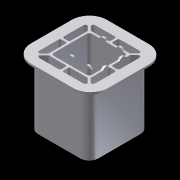
# Autodesk Inventor part: Part4
Saved by Autodesk Inventor 2012 (Build 160160000, 160)
## iProperties
Created: 2012-10-11
Part Number: Part4
Material: Default
Document SubType Name: Modeling
Designer: SONY
Density: 1 g/cm^3
Author: SONY
Autodesk Inventor part; units mm, degrees
ref_plane "YZ Plane" through (0, 0, 0) normal (1, 0, 0) x (0, 1, 0)
ref_plane "XZ Plane" through (0, 0, 0) normal (0, 1, 0) x (-1, 0, 0)
ref_plane "XY Plane" through (0, 0, 0) normal (0, 0, 1) x (1, 0, 0)
sketch "Sketch1" plane through (0, 0, 0) normal (0, 0, 1) x (1, 0, 0)
  line L0 (-50.8, 30.4821) -> (-50.8, -23.4929) projected
  arc A0 (-50.8, -23.4929) -> (-47.625, -26.6679) centre (-47.625, -23.4929) ccw projected
  line L1 (-47.625, -26.6679) -> (47.625, -26.6679) projected
  arc A1 (47.625, -26.6679) -> (50.8, -23.4929) centre (47.625, -23.4929) ccw projected
  line L2 (50.8, -23.4929) -> (50.8, 30.4821) projected
  line L3 (50.8, 30.4821) -> (25.4, 30.4821) projected
  line L4 (25.4, 30.4821) -> (25.4, 1.9071) projected
  arc A2 (22.225, -1.2679) -> (25.4, 1.9071) centre (22.225, 1.9071) ccw projected
  line L5 (22.225, -1.2679) -> (-22.225, -1.2679) projected
  arc A3 (-25.4, 1.9071) -> (-22.225, -1.2679) centre (-22.225, 1.9071) ccw projected
  line L6 (-25.4, 1.9071) -> (-25.4, 30.4821) projected
  line L7 (-25.4, 30.4821) -> (-50.8, 30.4821) projected
  arc A4 (-47.625, 87.6321) -> (-50.8, 84.4571) centre (-47.625, 84.4571) ccw projected
  line L8 (-50.8, 30.4821) -> (-50.8, 84.4571) projected
  line L9 (-25.4, 30.4821) -> (-50.8, 30.4821) projected
  line L10 (-25.4, 59.0571) -> (-25.4, 30.4821) projected
  arc A5 (-22.225, 62.2321) -> (-25.4, 59.0571) centre (-22.225, 59.0571) ccw projected
  line L11 (22.225, 62.2321) -> (-22.225, 62.2321) projected
  arc A6 (25.4, 59.0571) -> (22.225, 62.2321) centre (22.225, 59.0571) ccw projected
  line L12 (25.4, 30.4821) -> (25.4, 59.0571) projected
  line L13 (50.8, 30.4821) -> (25.4, 30.4821) projected
  line L14 (50.8, 84.4571) -> (50.8, 30.4821) projected
  arc A7 (50.8, 84.4571) -> (47.625, 87.6321) centre (47.625, 84.4571) ccw projected
  line L15 (-47.625, 87.6321) -> (47.625, 87.6321) projected
  line L16 (21.015, 0.6371) -> (19.215, 0.6371)
  line L17 (19.215, 0.6371) -> (19.215, 60.3271)
  line L18 (19.215, 60.3271) -> (21.015, 60.3271)
  line L19 (21.015, 60.3271) -> (21.015, 0.6371)
  line L20 (55.185, 0.6371) -> (56.985, 0.6371)
  line L21 (56.985, 0.6371) -> (56.985, 60.3271)
  line L22 (56.985, 60.3271) -> (55.185, 60.3271)
  line L23 (55.185, 60.3271) -> (55.185, 0.6371)
  line L24 (25.1349, 0.6371) -> (23.0176, 0.6371)
  line L25 (25.1349, 60.3271) -> (25.3032, 60.3271)
  line L26 (26.765, 60.3271) -> (23.1302, 60.3271) projected
  line L27 (23.015, 60.3271) -> (23.015, 0.6371) projected
  line L28 (53.185, -14.6029) -> (53.185, 64.1371) projected
  point P0 (0, 0)
  dimension "d0" = 1.8
  dimension "d1" = 1.8
  dimension "d34" = 59.69
  dimension "d115" = 2
  dimension "d116" = 2
  constraints: 20 end point, 4 collinear, 4 horizontal, 4 parallel, 2 perpendicular, 2 point on circle, 3 other
  measures "d0" distance between parallel lines of L23 L21
  measures "d1" distance of L17.end L18.end
  measures "d34" distance of L20.end L21.end
  measures "d115" distance between parallel lines of L27 L19
  measures "d116" distance between parallel lines of L23 L28
extrude "center_a" add sketch "Sketch1" against normal blind 25.4 contours L16 L17 L18 L19 | L23 L22 L21 L20
sketch "Sketch2" plane through (0, 0, 0) normal (0, 0, 1) x (1, 0, 0)
  line L0 (55.185, 0.6371) -> (56.985, 0.6371) projected
  line L1 (56.985, 0.6371) -> (56.985, 60.3271) projected
  line L2 (56.985, 60.3271) -> (55.185, 60.3271) projected
  line L3 (55.185, 60.3271) -> (55.185, 0.6371) projected
  line L4 (21.015, 0.6371) -> (19.215, 0.6371) projected
  line L5 (21.015, 60.3271) -> (21.015, 0.6371) projected
  line L6 (19.215, 60.3271) -> (21.015, 60.3271) projected
  line L7 (19.215, 0.6371) -> (19.215, 60.3271) projected
  arc A0 (-47.625, 87.6321) -> (-50.8, 84.4571) centre (-47.625, 84.4571) ccw projected
  line L8 (-50.8, 30.4821) -> (-50.8, 84.4571) projected
  line L9 (-25.4, 30.4821) -> (-50.8, 30.4821) projected
  line L10 (-25.4, 59.0571) -> (-25.4, 30.4821) projected
  arc A1 (-22.225, 62.2321) -> (-25.4, 59.0571) centre (-22.225, 59.0571) ccw projected
  line L11 (22.225, 62.2321) -> (-22.225, 62.2321) projected
  arc A2 (25.4, 59.0571) -> (22.225, 62.2321) centre (22.225, 59.0571) ccw projected
  line L12 (25.4, 30.4821) -> (25.4, 59.0571) projected
  line L13 (50.8, 30.4821) -> (25.4, 30.4821) projected
  line L14 (50.8, 84.4571) -> (50.8, 30.4821) projected
  arc A3 (50.8, 84.4571) -> (47.625, 87.6321) centre (47.625, 84.4571) ccw projected
  line L15 (-47.625, 87.6321) -> (47.625, 87.6321) projected
  line L16 (-50.8, 30.4821) -> (-50.8, -23.4929) projected
  arc A4 (-50.8, -23.4929) -> (-47.625, -26.6679) centre (-47.625, -23.4929) ccw projected
  line L17 (-47.625, -26.6679) -> (47.625, -26.6679) projected
  arc A5 (47.625, -26.6679) -> (50.8, -23.4929) centre (47.625, -23.4929) ccw projected
  line L18 (50.8, -23.4929) -> (50.8, 30.4821) projected
  line L19 (50.8, 30.4821) -> (25.4, 30.4821) projected
  line L20 (25.4, 30.4821) -> (25.4, 1.9071) projected
  arc A6 (22.225, -1.2679) -> (25.4, 1.9071) centre (22.225, 1.9071) ccw projected
  line L21 (22.225, -1.2679) -> (-22.225, -1.2679) projected
  arc A7 (-25.4, 1.9071) -> (-22.225, -1.2679) centre (-22.225, 1.9071) ccw projected
  line L22 (-25.4, 1.9071) -> (-25.4, 30.4821) projected
  line L23 (-25.4, 30.4821) -> (-50.8, 30.4821) projected
  point P0 (0, 0)
extrude "center_b" add sketch "Sketch2" along normal blind 4.4525 contours L3 L2 L1 L0 | L4 L7 L6 L5
sketch "Sketch3" plane through (0, 0, -25.4) normal (0, 0, -1) x (-1, 0, 0)
  line L0 (-21.015, 0.6371) -> (-21.015, 60.3271) projected
  line L1 (-19.215, 0.6371) -> (-21.015, 0.6371) projected
  line L2 (-19.215, 60.3271) -> (-19.215, 0.6371) projected
  line L3 (-21.015, 60.3271) -> (-19.215, 60.3271) projected
  line L4 (-56.985, 0.6371) -> (-56.985, 60.3271) projected
  line L5 (-55.185, 0.6371) -> (-56.985, 0.6371) projected
  line L6 (-55.185, 60.3271) -> (-55.185, 0.6371) projected
  line L7 (-56.985, 60.3271) -> (-55.185, 60.3271) projected
  point P0 (0, 0)
extrude "center_c" add sketch "Sketch3" along normal blind 4.4525
sketch "Sketch4" plane through (0, 0, -29.8525) normal (0, 0, -1) x (-1, 0, 0)
  line L0 (-56.985, 60.3271) -> (-55.185, 60.3271) projected
  line L1 (-56.985, 0.6371) -> (-56.985, 60.3271) projected
  line L2 (-55.185, 0.6371) -> (-56.985, 0.6371) projected
  line L3 (-55.185, 60.3271) -> (-55.185, 0.6371) projected
  line L4 (-56.985, 60.3271) -> (-19.215, 60.3271)
  line L5 (-19.215, 60.3271) -> (-19.215, 0.6371)
  line L6 (-19.215, 0.6371) -> (-56.985, 0.6371)
  line L7 (-56.985, 0.6371) -> (-56.985, 60.3271)
  point P0 (0, 0)
  constraints: 8 end point, 2 parallel, 1 horizontal, 1 perpendicular
extrude "center_d" add sketch "Sketch4" along normal blind 1.8
sketch "Sketch5" plane through (0, 0, 4.4525) normal (0, 0, 1) x (1, 0, 0)
  line L0 (55.185, 0.6371) -> (55.185, 60.3271) projected
  line L1 (56.985, 0.6371) -> (55.185, 0.6371) projected
  line L2 (56.985, 60.3271) -> (56.985, 0.6371) projected
  line L3 (55.185, 60.3271) -> (56.985, 60.3271) projected
  line L4 (19.215, 60.3271) -> (56.985, 60.3271)
  line L5 (56.985, 60.3271) -> (56.985, 0.6371)
  line L6 (56.985, 0.6371) -> (19.215, 0.6371)
  line L7 (19.215, 0.6371) -> (19.215, 60.3271)
  point P0 (0, 0)
  constraints: 8 end point, 2 parallel, 1 horizontal, 1 perpendicular
extrude "center_e" add sketch "Sketch5" along normal blind 1.8
fillet "internal-fillet" radius 3 4 edges at (19.215, 30.4821, -31.6525) (56.985, 30.4821, -31.6525) (19.215, 30.4821, 6.2525) (56.985, 30.4821, 6.2525)
fillet "internal-fillet" radius 2.5 4 edges at (55.185, 30.4821, -29.8525) (55.185, 30.4821, 4.4525) (21.015, 30.4821, 4.4525) (21.015, 30.4821, -29.8525)
sketch "Sketch25" plane through (22.215, 0.6371, 6.2525) normal (0, -1, 0) x (1, 0, 0)
  arc A0 (34.77, -3) -> (31.77, 0) centre (31.77, -3) ccw projected
  line L0 (31.77, 0) -> (0, 0) projected
  arc A1 (0, 0) -> (-3, -3) centre (0, -3) ccw projected
  line L1 (-3, -3) -> (-3, -34.905) projected
  arc A2 (-3, -34.905) -> (0, -37.905) centre (0, -34.905) ccw projected
  line L2 (0, -37.905) -> (31.77, -37.905) projected
  arc A3 (31.77, -37.905) -> (34.77, -34.905) centre (31.77, -34.905) ccw projected
  line L3 (34.77, -34.905) -> (34.77, -3) projected
  line L4 (1.3, -1.8) -> (30.47, -1.8) projected
  line L5 (-3, 8.15) -> (34.77, 8.15)
  line L6 (42.92, 0) -> (42.92, -37.905)
  line L7 (34.77, -46.055) -> (-3, -46.055)
  line L8 (-11.15, -37.905) -> (-11.15, 0)
  line L9 (-3, 0) -> (34.77, 0) construction
  line L10 (34.77, 0) -> (34.77, -37.905) construction
  line L11 (34.77, -37.905) -> (-3, -37.905) construction
  line L12 (-3, -37.905) -> (-3, 0) construction
  arc A4 (-3, 8.15) -> (-11.15, 0) centre (-3, 0) ccw
  arc A5 (-11.15, -37.905) -> (-3, -46.055) centre (-3, -37.905) ccw
  arc A6 (34.77, -46.055) -> (42.92, -37.905) centre (34.77, -37.905) ccw
  arc A7 (42.92, 0) -> (34.77, 8.15) centre (34.77, 0) ccw
  line L13 (34.77, 0) -> (-3, -37.905) construction
  line L14 (34.77, -37.905) -> (-3, 0) construction
  line L15 (16.5203, -18.315) -> (-8.0799, 6.3731) construction
  line L16 (15.2497, -19.59) -> (-9.355, 5.1026) construction
  line L17 (15.2497, -19.59) -> (39.8499, -44.2781) construction
  line L18 (16.5203, -18.315) -> (41.125, -43.0076) construction
  line L19 (-9.355, -43.0076) -> (39.8499, 6.3731) construction
  line L20 (41.125, 5.1026) -> (-8.0799, -44.2781) construction
  line L21 (39.8444, -41.7225) -> (34.4312, -36.2899)
  line L22 (38.5693, -42.993) -> (33.1595, -37.5638)
  line L23 (-6.7993, -42.993) -> (-1.3895, -37.5638)
  line L24 (-8.0744, -41.7225) -> (-2.6612, -36.2899)
  line L25 (-2.6612, -1.6151) -> (-8.0744, 3.8175)
  line L26 (-6.7993, 5.088) -> (-1.3895, -0.3412)
  line L27 (33.1595, -0.3412) -> (38.5693, 5.088)
  line L28 (39.8444, 3.8175) -> (34.4312, -1.6151)
  line L29 (15.885, -18.9525) -> (55.6698, -18.9525) construction
  line L30 (15.885, -18.9525) -> (-18.4202, -18.9525) construction
  line L31 (15.885, -18.9525) -> (15.885, 6.5335) construction
  line L32 (15.885, -18.9525) -> (15.885, -60.1449) construction
  line L33 (14.985, 22.3974) -> (16.785, 22.3974) construction
  line L34 (16.785, 22.3974) -> (16.785, -69.4541) construction
  line L35 (16.785, -69.4541) -> (14.985, -69.4541) construction
  line L36 (14.985, -69.4541) -> (14.985, 22.3974) construction
  line L37 (64.878, -19.8525) -> (-35.3195, -19.8525) construction
  line L38 (-35.3195, -19.8525) -> (-35.3195, -18.0525) construction
  line L39 (-35.3195, -18.0525) -> (64.878, -18.0525) construction
  line L40 (64.878, -18.0525) -> (64.878, -19.8525) construction
  line L41 (34.77, -18.0525) -> (41.12, -18.0525)
  line L42 (41.12, -19.8525) -> (34.77, -19.8525)
  line L43 (16.785, 0) -> (16.785, 6.35)
  line L44 (14.985, 6.35) -> (14.985, 0)
  line L45 (-3, -18.0525) -> (-9.35, -18.0525)
  line L46 (-9.35, -19.8525) -> (-3, -19.8525)
  line L47 (16.785, -37.905) -> (16.785, -44.255)
  line L48 (14.985, -44.255) -> (14.985, -37.905)
  line L49 (41.12, 0) -> (41.12, -18.0525)
  line L50 (41.12, -19.8525) -> (41.12, -37.905)
  line L51 (-9.35, -37.905) -> (-9.35, -19.8525)
  line L52 (-9.35, -18.0525) -> (-9.35, 0)
  line L53 (34.77, -44.255) -> (16.785, -44.255)
  line L54 (14.985, -44.255) -> (-3, -44.255)
  arc A8 (34.77, -44.255) -> (38.5693, -42.993) centre (34.77, -37.905) ccw
  arc A9 (39.8444, -41.7225) -> (41.12, -37.905) centre (34.77, -37.905) ccw
  arc A10 (-9.35, -37.905) -> (-8.0744, -41.7225) centre (-3, -37.905) ccw
  arc A11 (-6.7993, -42.993) -> (-3, -44.255) centre (-3, -37.905) ccw
  arc A12 (41.12, 0) -> (39.8444, 3.8175) centre (34.77, 0) ccw
  arc A13 (38.5693, 5.088) -> (34.77, 6.35) centre (34.77, 0) ccw
  line L55 (-3, 6.35) -> (14.985, 6.35)
  line L56 (16.785, 6.35) -> (34.77, 6.35)
  arc A14 (-3, 6.35) -> (-6.7993, 5.088) centre (-3, 0) ccw
  arc A15 (-8.0744, 3.8175) -> (-9.35, 0) centre (-3, 0) ccw
  line L57 (-3, -18.0525) -> (-3, -19.8525)
  line L58 (14.985, 0) -> (16.785, 0)
  line L59 (34.77, -18.0525) -> (34.77, -19.8525)
  line L60 (16.785, -37.905) -> (14.985, -37.905)
  line L61 (19.3458, 41.1317) -> (44.9845, 41.1317) construction
  line L62 (44.9845, 41.1317) -> (44.9845, 37.9997) construction
  line L63 (44.9845, 37.9997) -> (19.3458, 37.9997) construction
  line L64 (19.3458, 37.9997) -> (19.3458, 41.1317) construction
  dimension "d166" = 1.8
  dimension "d171" = 0.9
  dimension "d172" = 1.8
  dimension "d173" = 1.8
  dimension "d174" = 0.9
  dimension "d175" = 0.9
  dimension "d176" = 0.9
  dimension "d177" = 0.9
  dimension "d178" = 1.8
  dimension "d179" = 1.8
  dimension "d180" = 1.8
  dimension "d181" = 6.35
  dimension "d182" = 6.35
  dimension "d183" = 6.35
  constraints: 112 end point, 42 point on line, 40 point on circle, 23 parallel, 22 tangent, 12 centre point, 10 collinear, 10 perpendicular, 8 coincident, 6 horizontal, 1 midpoint, 2 other
  measures "d166" distance between parallel lines of L4 L0
  measures "d171" distance between parallel lines of L15 L14
  measures "d172" distance between parallel lines of L16 L15
  measures "d173" distance between parallel lines of L19 L20
  measures "d174" distance between parallel lines of L13 L19
  measures "d175" distance between parallel lines of L32 L36
  measures "d176" distance between parallel lines of L32 L34
  measures "d177" distance between parallel lines of L29 L37
  measures "d178" distance between parallel lines of L37 L39
  measures "d179" radial gap between concentric circles of A5 A10
  measures "d180" distance between parallel lines of L54 L7
  measures "d181" distance between parallel lines of L55 L0
  measures "d182" distance between parallel lines of L1 L52
  measures "d183" distance between parallel lines of L49 L3
extrude "spiderweb" add sketch "Sketch25" against normal up to surface (59.69 mm away)
sketch "Sketch26" plane through (19.215, 60.3271, 14.4025) normal (0, 1, 0) x (1, 0, 0)
  line L0 (0, -8.8849) -> (37.77, -8.8849)
  line L1 (56.08, 9.4251) -> (56.08, 46.055)
  line L2 (37.77, 64.365) -> (0, 64.365)
  line L3 (-18.31, 46.055) -> (-18.31, 9.4251)
  arc A0 (-18.31, 9.4251) -> (0, -8.8849) centre (0, 9.4251) ccw
  arc A1 (37.77, -8.8849) -> (56.08, 9.4251) centre (37.77, 9.4251) ccw
  arc A2 (56.08, 46.055) -> (37.77, 64.365) centre (37.77, 46.055) ccw
  arc A3 (0, 64.365) -> (-18.31, 46.055) centre (0, 46.055) ccw
  arc A4 (37.4312, 9.7651) -> (37.77, 11.15) centre (34.77, 11.15) ccw projected
  line L4 (37.77, 26.2025) -> (37.77, 11.15) projected
  line L5 (44.12, 26.2025) -> (37.77, 26.2025) projected
  line L6 (44.12, 8.15) -> (44.12, 26.2025) projected
  arc A5 (42.8444, 4.3325) -> (44.12, 8.15) centre (37.77, 8.15) ccw projected
  line L7 (37.4312, 9.7651) -> (42.8444, 4.3325) projected
  line L8 (37.77, 43.055) -> (37.77, 28.0025) projected
  arc A6 (37.77, 43.055) -> (37.4312, 44.4399) centre (34.77, 43.055) ccw projected
  line L9 (42.8444, 49.8725) -> (37.4312, 44.4399) projected
  arc A7 (44.12, 46.055) -> (42.8444, 49.8725) centre (37.77, 46.055) ccw projected
  line L10 (44.12, 28.0025) -> (44.12, 46.055) projected
  line L11 (37.77, 28.0025) -> (44.12, 28.0025) projected
  arc A8 (36.1595, 45.7138) -> (34.77, 46.055) centre (34.77, 43.055) ccw projected
  line L12 (34.77, 46.055) -> (19.785, 46.055) projected
  line L13 (19.785, 52.405) -> (19.785, 46.055) projected
  line L14 (37.77, 52.405) -> (19.785, 52.405) projected
  arc A9 (41.5693, 51.143) -> (37.77, 52.405) centre (37.77, 46.055) ccw projected
  line L15 (36.1595, 45.7138) -> (41.5693, 51.143) projected
  line L16 (17.985, 46.055) -> (3, 46.055) projected
  arc A10 (3, 46.055) -> (1.6105, 45.7138) centre (3, 43.055) ccw projected
  line L17 (-3.7993, 51.143) -> (1.6105, 45.7138) projected
  arc A11 (0, 52.405) -> (-3.7993, 51.143) centre (0, 46.055) ccw projected
  line L18 (17.985, 52.405) -> (0, 52.405) projected
  line L19 (17.985, 46.055) -> (17.985, 52.405) projected
  line L20 (0, 11.15) -> (0, 26.2025) projected
  arc A12 (0, 11.15) -> (0.3388, 9.7651) centre (3, 11.15) ccw projected
  line L21 (-5.0744, 4.3325) -> (0.3388, 9.7651) projected
  arc A13 (-6.35, 8.15) -> (-5.0744, 4.3325) centre (0, 8.15) ccw projected
  line L22 (-6.35, 26.2025) -> (-6.35, 8.15) projected
  line L23 (0, 26.2025) -> (-6.35, 26.2025) projected
  line L24 (-6.35, 28.0025) -> (0, 28.0025) projected
  line L25 (-6.35, 46.055) -> (-6.35, 28.0025) projected
  arc A14 (-5.0744, 49.8725) -> (-6.35, 46.055) centre (0, 46.055) ccw projected
  line L26 (0.3388, 44.4399) -> (-5.0744, 49.8725) projected
  arc A15 (0.3388, 44.4399) -> (0, 43.055) centre (3, 43.055) ccw projected
  line L27 (0, 28.0025) -> (0, 43.055) projected
  arc A16 (1.6105, 8.4912) -> (3, 8.15) centre (3, 11.15) ccw projected
  line L28 (3, 8.15) -> (17.985, 8.15) projected
  line L29 (17.985, 1.8) -> (17.985, 8.15) projected
  line L30 (0, 1.8) -> (17.985, 1.8) projected
  arc A17 (-3.7993, 3.062) -> (0, 1.8) centre (0, 8.15) ccw projected
  line L31 (1.6105, 8.4912) -> (-3.7993, 3.062) projected
  arc A18 (-8.15, 8.15) -> (0, 0) centre (0, 8.15) ccw projected
  line L32 (37.77, 0) -> (0, 0) projected
  arc A19 (37.77, 0) -> (45.92, 8.15) centre (37.77, 8.15) ccw projected
  line L33 (45.92, 46.055) -> (45.92, 8.15) projected
  arc A20 (45.92, 46.055) -> (37.77, 54.205) centre (37.77, 46.055) ccw projected
  line L34 (0, 54.205) -> (37.77, 54.205) projected
  arc A21 (0, 54.205) -> (-8.15, 46.055) centre (0, 46.055) ccw projected
  line L35 (-8.15, 8.15) -> (-8.15, 46.055) projected
  line L36 (41.5693, 3.062) -> (36.1595, 8.4912) projected
  arc A22 (37.77, 1.8) -> (41.5693, 3.062) centre (37.77, 8.15) ccw projected
  line L37 (19.785, 1.8) -> (37.77, 1.8) projected
  line L38 (19.785, 8.15) -> (19.785, 1.8) projected
  line L39 (19.785, 8.15) -> (34.77, 8.15) projected
  arc A23 (34.77, 8.15) -> (36.1595, 8.4912) centre (34.77, 11.15) ccw projected
  line L40 (33.47, 9.95) -> (4.3, 9.95) projected
  arc A24 (1.8, 12.45) -> (4.3, 9.95) centre (4.3, 12.45) ccw projected
  line L41 (1.8, 12.45) -> (1.8, 41.755) projected
  arc A25 (4.3, 44.255) -> (1.8, 41.755) centre (4.3, 41.755) ccw projected
  line L42 (4.3, 44.255) -> (33.47, 44.255) projected
  arc A26 (35.97, 41.755) -> (33.47, 44.255) centre (33.47, 41.755) ccw projected
  line L43 (35.97, 41.755) -> (35.97, 12.45) projected
  arc A27 (33.47, 9.95) -> (35.97, 12.45) centre (33.47, 12.45) ccw projected
  dimension "d206" = 10.16
  constraints: 8 end point, 8 point on circle, 8 tangent, 4 centre point, 3 perpendicular, 2 coincident, 2 horizontal alignment, 2 vertical alignment, 1 point on line
  measures "d206" distance between parallel lines of L2 L34
extrude "flat base" add sketch "Sketch26" against normal blind 1.8 contours A0 L3 A3 L2 A2 L1 A1 L0
fillet "superfillet" radius 1.5 40 edges at (60.7843, 30.4821, 11.3405) (62.0594, 30.4821, 10.07) (63.335, 30.4821, -11.8) (63.335, 30.4821, -13.6) (62.0594, 30.4821, -35.47) (60.7843, 30.4821, -36.7405) (39, 30.4821, -38.0025) (37.2, 30.4821, -38.0025) (14.1406, 30.4821, 10.07) (12.865, 30.4821, -11.8) (12.865, 30.4821, -13.6) (14.1406, 30.4821, -35.47) (39, 30.4821, 12.6025) (37.2, 30.4821, 12.6025) (15.4157, 30.4821, 11.3405) (15.4157, 30.4821, -36.7405) (19.215, 30.4821, -11.8) (20.8255, 30.4821, 5.9113) (55.3745, 30.4821, 5.9113) (56.985, 30.4821, -11.8) (56.6462, 30.4821, 4.6374) (39, 30.4821, 6.2525) (19.215, 30.4821, -13.6) (20.8255, 30.4821, -31.3113) (19.5538, 30.4821, -30.0374) (39, 30.4821, -31.6525) (37.2, 30.4821, -31.6525) (56.6462, 30.4821, -30.0374) (56.985, 30.4821, -13.6) (55.3745, 30.4821, -31.3113) (13.4521, 58.5271, 12.0154) (11.065, 58.5271, -12.7) (13.4521, 58.5271, -37.4154) (38.1, 58.5271, -39.8025) (62.7479, 58.5271, -37.4154) (65.135, 58.5271, -12.7) (62.7479, 58.5271, 12.0154) (38.1, 58.5271, 14.4025) (37.2, 30.4821, 6.2525) (19.5538, 30.4821, 4.6374)
sketch "Sketch27" plane through (19.215, 0.6371, 14.4025) normal (0, -1, 0) x (1, 0, 0)
  arc A0 (35.4337, -8.2243) -> (34.77, -8.15) centre (34.77, -11.15) ccw projected
  line L0 (34.77, -8.15) -> (21.285, -8.15) projected
  arc A1 (19.785, -6.65) -> (21.285, -8.15) centre (21.285, -6.65) ccw projected
  line L1 (19.785, -6.65) -> (19.785, -3.3) projected
  arc A2 (21.285, -1.8) -> (19.785, -3.3) centre (21.285, -3.3) ccw projected
  line L2 (21.285, -1.8) -> (37.77, -1.8) projected
  arc A3 (39.439, -2.0233) -> (37.77, -1.8) centre (37.77, -8.15) ccw projected
  arc A4 (40.1073, -4.5293) -> (39.439, -2.0233) centre (39.0447, -3.4705) ccw projected
  line L3 (40.1073, -4.5293) -> (36.828, -7.8203) projected
  arc A5 (35.4337, -8.2243) -> (36.828, -7.8203) centre (35.7655, -6.7615) ccw projected
  line L4 (38.0964, -9.0975) -> (41.3824, -5.7998) projected
  arc A6 (43.8907, -6.4592) -> (41.3824, -5.7998) centre (42.4449, -6.8586) ccw projected
  arc A7 (44.12, -8.15) -> (43.8907, -6.4592) centre (37.77, -8.15) ccw projected
  line L5 (44.12, -8.15) -> (44.12, -24.7025) projected
  arc A8 (42.62, -26.2025) -> (44.12, -24.7025) centre (42.62, -24.7025) ccw projected
  line L6 (42.62, -26.2025) -> (39.27, -26.2025) projected
  arc A9 (37.77, -24.7025) -> (39.27, -26.2025) centre (39.27, -24.7025) ccw projected
  line L7 (37.77, -24.7025) -> (37.77, -11.15) projected
  arc A10 (37.77, -11.15) -> (37.6959, -10.4875) centre (34.77, -11.15) ccw projected
  arc A11 (38.0964, -9.0975) -> (37.6959, -10.4875) centre (39.1589, -10.1563) ccw projected
  line L8 (39.27, -28.0025) -> (42.62, -28.0025) projected
  arc A12 (44.12, -29.5025) -> (42.62, -28.0025) centre (42.62, -29.5025) ccw projected
  line L9 (44.12, -29.5025) -> (44.12, -46.055) projected
  arc A13 (43.8907, -47.7458) -> (44.12, -46.055) centre (37.77, -46.055) ccw projected
  arc A14 (41.3824, -48.4052) -> (43.8907, -47.7458) centre (42.4449, -47.3464) ccw projected
  line L10 (41.3824, -48.4052) -> (38.0964, -45.1075) projected
  arc A15 (37.6959, -43.7175) -> (38.0964, -45.1075) centre (39.1589, -44.0487) ccw projected
  arc A16 (37.6959, -43.7175) -> (37.77, -43.055) centre (34.77, -43.055) ccw projected
  line L11 (37.77, -43.055) -> (37.77, -29.5025) projected
  arc A17 (39.27, -28.0025) -> (37.77, -29.5025) centre (39.27, -29.5025) ccw projected
  line L12 (36.828, -46.3847) -> (40.1073, -49.6757) projected
  arc A18 (39.439, -52.1817) -> (40.1073, -49.6757) centre (39.0447, -50.7345) ccw projected
  arc A19 (37.77, -52.405) -> (39.439, -52.1817) centre (37.77, -46.055) ccw projected
  line L13 (37.77, -52.405) -> (21.285, -52.405) projected
  arc A20 (19.785, -50.905) -> (21.285, -52.405) centre (21.285, -50.905) ccw projected
  line L14 (19.785, -50.905) -> (19.785, -47.555) projected
  arc A21 (21.285, -46.055) -> (19.785, -47.555) centre (21.285, -47.555) ccw projected
  line L15 (21.285, -46.055) -> (34.77, -46.055) projected
  arc A22 (34.77, -46.055) -> (35.4337, -45.9807) centre (34.77, -43.055) ccw projected
  arc A23 (36.828, -46.3847) -> (35.4337, -45.9807) centre (35.7655, -47.4435) ccw projected
  line L16 (0, -29.5025) -> (0, -43.055) projected
  arc A24 (0, -43.055) -> (0.0741, -43.7175) centre (3, -43.055) ccw projected
  arc A25 (-0.3264, -45.1075) -> (0.0741, -43.7175) centre (-1.3889, -44.0487) ccw projected
  line L17 (-0.3264, -45.1075) -> (-3.6124, -48.4052) projected
  arc A26 (-6.1207, -47.7458) -> (-3.6124, -48.4052) centre (-4.6749, -47.3464) ccw projected
  arc A27 (-6.35, -46.055) -> (-6.1207, -47.7458) centre (0, -46.055) ccw projected
  line L18 (-6.35, -46.055) -> (-6.35, -29.5025) projected
  arc A28 (-4.85, -28.0025) -> (-6.35, -29.5025) centre (-4.85, -29.5025) ccw projected
  line L19 (-4.85, -28.0025) -> (-1.5, -28.0025) projected
  arc A29 (0, -29.5025) -> (-1.5, -28.0025) centre (-1.5, -29.5025) ccw projected
  line L20 (17.985, -47.555) -> (17.985, -50.905) projected
  arc A30 (16.485, -52.405) -> (17.985, -50.905) centre (16.485, -50.905) ccw projected
  line L21 (16.485, -52.405) -> (0, -52.405) projected
  arc A31 (-1.669, -52.1817) -> (0, -52.405) centre (0, -46.055) ccw projected
  arc A32 (-2.3373, -49.6757) -> (-1.669, -52.1817) centre (-1.2747, -50.7345) ccw projected
  line L22 (-2.3373, -49.6757) -> (0.942, -46.3847) projected
  arc A33 (2.3363, -45.9807) -> (0.942, -46.3847) centre (2.0045, -47.4435) ccw projected
  arc A34 (2.3363, -45.9807) -> (3, -46.055) centre (3, -43.055) ccw projected
  line L23 (3, -46.055) -> (16.485, -46.055) projected
  arc A35 (17.985, -47.555) -> (16.485, -46.055) centre (16.485, -47.555) ccw projected
  line L24 (0, 0) -> (37.77, 0) projected
  arc A36 (0, 0) -> (-8.15, -8.15) centre (0, -8.15) ccw projected
  line L25 (-8.15, -46.055) -> (-8.15, -8.15) projected
  arc A37 (-8.15, -46.055) -> (0, -54.205) centre (0, -46.055) ccw projected
  line L26 (37.77, -54.205) -> (0, -54.205) projected
  arc A38 (37.77, -54.205) -> (45.92, -46.055) centre (37.77, -46.055) ccw projected
  line L27 (45.92, -8.15) -> (45.92, -46.055) projected
  arc A39 (45.92, -8.15) -> (37.77, 0) centre (37.77, -8.15) ccw projected
  line L28 (35.97, -12.45) -> (35.97, -41.755) projected
  arc A40 (33.47, -44.255) -> (35.97, -41.755) centre (33.47, -41.755) ccw projected
  line L29 (33.47, -44.255) -> (4.3, -44.255) projected
  arc A41 (1.8, -41.755) -> (4.3, -44.255) centre (4.3, -41.755) ccw projected
  line L30 (1.8, -41.755) -> (1.8, -12.45) projected
  arc A42 (4.3, -9.95) -> (1.8, -12.45) centre (4.3, -12.45) ccw projected
  line L31 (4.3, -9.95) -> (33.47, -9.95) projected
  arc A43 (35.97, -12.45) -> (33.47, -9.95) centre (33.47, -12.45) ccw projected
  arc A44 (35.4337, -8.2243) -> (34.77, -8.15) centre (34.77, -11.15) ccw projected
  line L32 (34.77, -8.15) -> (21.285, -8.15) projected
  arc A45 (19.785, -6.65) -> (21.285, -8.15) centre (21.285, -6.65) ccw projected
  line L33 (19.785, -6.65) -> (19.785, -3.3) projected
  line L34 (40.1073, -4.5293) -> (36.828, -7.8203) projected
  arc A46 (35.4337, -8.2243) -> (36.828, -7.8203) centre (35.7655, -6.7615) ccw projected
  line L35 (38.0964, -9.0975) -> (41.3824, -5.7998) projected
  line L36 (42.62, -26.2025) -> (39.27, -26.2025) projected
  arc A47 (37.77, -24.7025) -> (39.27, -26.2025) centre (39.27, -24.7025) ccw projected
  line L37 (37.77, -24.7025) -> (37.77, -11.15) projected
  arc A48 (37.77, -11.15) -> (37.6959, -10.4875) centre (34.77, -11.15) ccw projected
  arc A49 (38.0964, -9.0975) -> (37.6959, -10.4875) centre (39.1589, -10.1563) ccw projected
  line L38 (39.27, -28.0025) -> (42.62, -28.0025) projected
  line L39 (41.3824, -48.4052) -> (38.0964, -45.1075) projected
  arc A50 (37.6959, -43.7175) -> (38.0964, -45.1075) centre (39.1589, -44.0487) ccw projected
  arc A51 (37.6959, -43.7175) -> (37.77, -43.055) centre (34.77, -43.055) ccw projected
  line L40 (37.77, -43.055) -> (37.77, -29.5025) projected
  arc A52 (39.27, -28.0025) -> (37.77, -29.5025) centre (39.27, -29.5025) ccw projected
  line L41 (36.828, -46.3847) -> (40.1073, -49.6757) projected
  arc A53 (39.439, -52.1817) -> (40.1073, -49.6757) centre (39.0447, -50.7345) ccw projected
  arc A54 (37.77, -52.405) -> (39.439, -52.1817) centre (37.77, -46.055) ccw projected
  line L42 (37.77, -52.405) -> (21.285, -52.405) projected
  arc A55 (19.785, -50.905) -> (21.285, -52.405) centre (21.285, -50.905) ccw projected
  line L43 (19.785, -50.905) -> (19.785, -47.555) projected
  arc A56 (21.285, -46.055) -> (19.785, -47.555) centre (21.285, -47.555) ccw projected
  line L44 (21.285, -46.055) -> (34.77, -46.055) projected
  arc A57 (34.77, -46.055) -> (35.4337, -45.9807) centre (34.77, -43.055) ccw projected
  arc A58 (36.828, -46.3847) -> (35.4337, -45.9807) centre (35.7655, -47.4435) ccw projected
  line L45 (0, -29.5025) -> (0, -43.055) projected
  arc A59 (0, -43.055) -> (0.0741, -43.7175) centre (3, -43.055) ccw projected
  arc A60 (-0.3264, -45.1075) -> (0.0741, -43.7175) centre (-1.3889, -44.0487) ccw projected
  line L46 (-0.3264, -45.1075) -> (-3.6124, -48.4052) projected
  arc A61 (-6.1207, -47.7458) -> (-3.6124, -48.4052) centre (-4.6749, -47.3464) ccw projected
  arc A62 (-6.35, -46.055) -> (-6.1207, -47.7458) centre (0, -46.055) ccw projected
  line L47 (-6.35, -46.055) -> (-6.35, -29.5025) projected
  arc A63 (-4.85, -28.0025) -> (-6.35, -29.5025) centre (-4.85, -29.5025) ccw projected
  line L48 (-4.85, -28.0025) -> (-1.5, -28.0025) projected
  arc A64 (0, -29.5025) -> (-1.5, -28.0025) centre (-1.5, -29.5025) ccw projected
  line L49 (17.985, -47.555) -> (17.985, -50.905) projected
  arc A65 (16.485, -52.405) -> (17.985, -50.905) centre (16.485, -50.905) ccw projected
  line L50 (16.485, -52.405) -> (0, -52.405) projected
  arc A66 (-1.669, -52.1817) -> (0, -52.405) centre (0, -46.055) ccw projected
  arc A67 (-2.3373, -49.6757) -> (-1.669, -52.1817) centre (-1.2747, -50.7345) ccw projected
  line L51 (-2.3373, -49.6757) -> (0.942, -46.3847) projected
  arc A68 (2.3363, -45.9807) -> (0.942, -46.3847) centre (2.0045, -47.4435) ccw projected
  arc A69 (2.3363, -45.9807) -> (3, -46.055) centre (3, -43.055) ccw projected
  line L52 (3, -46.055) -> (16.485, -46.055) projected
  arc A70 (17.985, -47.555) -> (16.485, -46.055) centre (16.485, -47.555) ccw projected
  line L53 (-1.5, -26.2025) -> (-4.85, -26.2025) projected
  arc A71 (-6.35, -24.7025) -> (-4.85, -26.2025) centre (-4.85, -24.7025) ccw projected
  line L54 (-6.35, -24.7025) -> (-6.35, -8.15) projected
  arc A72 (-6.1207, -6.4592) -> (-6.35, -8.15) centre (0, -8.15) ccw projected
  arc A73 (-3.6124, -5.7998) -> (-6.1207, -6.4592) centre (-4.6749, -6.8586) ccw projected
  line L55 (-3.6124, -5.7998) -> (-0.3264, -9.0975) projected
  arc A74 (0.0741, -10.4875) -> (-0.3264, -9.0975) centre (-1.3889, -10.1563) ccw projected
  arc A75 (0.0741, -10.4875) -> (0, -11.15) centre (3, -11.15) ccw projected
  line L56 (0, -11.15) -> (0, -24.7025) projected
  arc A76 (-1.5, -26.2025) -> (0, -24.7025) centre (-1.5, -24.7025) ccw projected
  line L57 (0, 0) -> (37.77, 0) projected
  arc A77 (0, 0) -> (-8.15, -8.15) centre (0, -8.15) ccw projected
  line L58 (-8.15, -46.055) -> (-8.15, -8.15) projected
  arc A78 (-8.15, -46.055) -> (0, -54.205) centre (0, -46.055) ccw projected
  line L59 (37.77, -54.205) -> (0, -54.205) projected
  arc A79 (37.77, -54.205) -> (45.92, -46.055) centre (37.77, -46.055) ccw projected
  line L60 (45.92, -8.15) -> (45.92, -46.055) projected
  arc A80 (45.92, -8.15) -> (37.77, 0) centre (37.77, -8.15) ccw projected
  line L61 (0.942, -7.8203) -> (-2.3373, -4.5293) projected
  line L62 (17.985, -3.3) -> (17.985, -6.65) projected
  arc A81 (16.485, -8.15) -> (17.985, -6.65) centre (16.485, -6.65) ccw projected
  line L63 (16.485, -8.15) -> (3, -8.15) projected
  arc A82 (3, -8.15) -> (2.3363, -8.2243) centre (3, -11.15) ccw projected
  arc A83 (0.942, -7.8203) -> (2.3363, -8.2243) centre (2.0045, -6.7615) ccw projected
  line L64 (35.97, -12.45) -> (35.97, -41.755) projected
  arc A84 (33.47, -44.255) -> (35.97, -41.755) centre (33.47, -41.755) ccw projected
  line L65 (33.47, -44.255) -> (4.3, -44.255) projected
  arc A85 (1.8, -41.755) -> (4.3, -44.255) centre (4.3, -41.755) ccw projected
  line L66 (1.8, -41.755) -> (1.8, -12.45) projected
  arc A86 (4.3, -9.95) -> (1.8, -12.45) centre (4.3, -12.45) ccw projected
  line L67 (4.3, -9.95) -> (33.47, -9.95) projected
  arc A87 (35.97, -12.45) -> (33.47, -9.95) centre (33.47, -12.45) ccw projected
  arc A88 (21.285, -1.8) -> (19.785, -3.3) centre (21.285, -3.3) ccw projected
  line L68 (21.285, -1.8) -> (37.77, -1.8) projected
  arc A89 (39.439, -2.0233) -> (37.77, -1.8) centre (37.77, -8.15) ccw projected
  arc A90 (40.1073, -4.5293) -> (39.439, -2.0233) centre (39.0447, -3.4705) ccw projected
  arc A91 (43.8907, -6.4592) -> (41.3824, -5.7998) centre (42.4449, -6.8586) ccw projected
  arc A92 (44.12, -8.15) -> (43.8907, -6.4592) centre (37.77, -8.15) ccw projected
  line L69 (44.12, -8.15) -> (44.12, -24.7025) projected
  arc A93 (42.62, -26.2025) -> (44.12, -24.7025) centre (42.62, -24.7025) ccw projected
  arc A94 (44.12, -29.5025) -> (42.62, -28.0025) centre (42.62, -29.5025) ccw projected
  line L70 (44.12, -29.5025) -> (44.12, -46.055) projected
  arc A95 (43.8907, -47.7458) -> (44.12, -46.055) centre (37.77, -46.055) ccw projected
  arc A96 (41.3824, -48.4052) -> (43.8907, -47.7458) centre (42.4449, -47.3464) ccw projected
  arc A97 (-1.669, -2.0233) -> (-2.3373, -4.5293) centre (-1.2747, -3.4705) ccw projected
  arc A98 (0, -1.8) -> (-1.669, -2.0233) centre (0, -8.15) ccw projected
  line L71 (0, -1.8) -> (16.485, -1.8) projected
  arc A99 (17.985, -3.3) -> (16.485, -1.8) centre (16.485, -3.3) ccw projected
  point P0 (0.3388, -13.5751)
  point P1 (17.985, -11.96)
  point P2 (-19.215, -14.4025)
  point P3 (47.19, -29.2725)
  point P4 (47.19, -27.4725)
  point P5 (45.0262, -3.413)
  point P6 (43.7511, -2.1424)
  point P7 (19.785, 0)
  point P8 (17.985, 0)
  point P9 (-5.9811, -2.1424)
  point P10 (45.0262, -53.332)
  constraints: 9 other
extrude "haircut" cut sketch "Sketch27" against normal blind 1.8 contours L24 A39 L27 A38 L26 A37 L25 A36 | L61 A97 A98 L71 A99 L62 A81 L63 A82 A83
sketch "Sketch28" plane through (19.215, 60.3271, 23.2874) normal (0, 1, 0) x (1, 0, 0)
  line L0 (37.77, 51.9399) -> (37.77, 38.3874) projected
  line L1 (34.77, 54.9399) -> (21.285, 54.9399) projected
  line L2 (16.485, 54.9399) -> (3, 54.9399) projected
  line L3 (4.3, 53.1399) -> (33.47, 53.1399) projected
  line L4 (35.97, 50.6399) -> (35.97, 21.3349) projected
  arc A0 (26.35, 54.9224) -> (23.85, 57.4224) centre (23.85, 54.9224) ccw projected
  line L5 (23.85, 57.4224) -> (18.69, 57.4224) projected
  arc A1 (18.69, 57.4224) -> (16.19, 54.9224) centre (18.69, 54.9224) ccw projected
  line L6 (16.19, 53.5724) -> (16.19, 54.9224) projected
  arc A2 (13.69, 51.0724) -> (16.19, 53.5724) centre (13.69, 53.5724) ccw projected
  line L7 (6.3, 51.0724) -> (13.69, 51.0724) projected
  line L8 (6.3, 49.3224) -> (6.3, 51.0724) projected
  line L9 (6.3, 49.3224) -> (30.22, 49.3224) projected
  arc A3 (32.22, 47.3224) -> (30.22, 49.3224) centre (30.22, 47.3224) ccw projected
  line L10 (32.22, 47.3224) -> (32.22, 24.6524) projected
  arc A4 (30.22, 22.6524) -> (32.22, 24.6524) centre (30.22, 24.6524) ccw projected
  line L11 (30.22, 22.6524) -> (6.3, 22.6524) projected
  line L12 (6.3, 20.9024) -> (6.3, 22.6524) projected
  line L13 (13.69, 20.9024) -> (6.3, 20.9024) projected
  arc A5 (16.19, 18.4024) -> (13.69, 20.9024) centre (13.69, 18.4024) ccw projected
  line L14 (16.19, 18.4024) -> (16.19, 17.0524) projected
  arc A6 (16.19, 17.0524) -> (18.69, 14.5524) centre (18.69, 17.0524) ccw projected
  line L15 (18.69, 14.5524) -> (23.85, 14.5524) projected
  arc A7 (23.85, 14.5524) -> (26.35, 17.0524) centre (23.85, 17.0524) ccw projected
  line L16 (26.35, 18.4024) -> (26.35, 17.0524) projected
  arc A8 (28.85, 20.9024) -> (26.35, 18.4024) centre (28.85, 18.4024) ccw projected
  line L17 (31.47, 20.9024) -> (28.85, 20.9024) projected
  arc A9 (31.47, 20.9024) -> (33.97, 23.4024) centre (31.47, 23.4024) ccw projected
  line L18 (33.97, 28.4074) -> (33.97, 23.4024) projected
  arc A10 (36.47, 30.9074) -> (33.97, 28.4074) centre (36.47, 28.4074) ccw projected
  line L19 (36.47, 30.9074) -> (37.82, 30.9074) projected
  arc A11 (37.82, 30.9074) -> (40.32, 33.4074) centre (37.82, 33.4074) ccw projected
  line L20 (40.32, 33.4074) -> (40.32, 38.5674) projected
  arc A12 (40.32, 38.5674) -> (37.82, 41.0674) centre (37.82, 38.5674) ccw projected
  line L21 (36.47, 41.0674) -> (37.82, 41.0674) projected
  arc A13 (33.97, 43.5674) -> (36.47, 41.0674) centre (36.47, 43.5674) ccw projected
  line L22 (33.97, 48.5724) -> (33.97, 43.5674) projected
  arc A14 (33.97, 48.5724) -> (31.47, 51.0724) centre (31.47, 48.5724) ccw projected
  line L23 (28.85, 51.0724) -> (31.47, 51.0724) projected
  arc A15 (26.35, 53.5724) -> (28.85, 51.0724) centre (28.85, 53.5724) ccw projected
  line L24 (26.35, 53.5724) -> (26.35, 54.9224) projected
  line L25 (10.71, 54.9399) -> (15.79, 54.9399)
  line L26 (15.79, 54.9399) -> (15.79, 53.1399)
  line L27 (15.79, 53.1399) -> (10.71, 53.1399)
  line L28 (10.71, 53.1399) -> (10.71, 54.9399)
  line L29 (26.75, 54.9399) -> (31.83, 54.9399)
  line L30 (31.83, 54.9399) -> (31.83, 53.1399)
  line L31 (31.83, 53.1399) -> (26.75, 53.1399)
  line L32 (26.75, 53.1399) -> (26.75, 54.9399)
  line L33 (35.97, 46.5474) -> (37.77, 46.5474)
  line L34 (37.77, 46.5474) -> (37.77, 41.4674)
  line L35 (37.77, 41.4674) -> (35.97, 41.4674)
  line L36 (35.97, 41.4674) -> (35.97, 46.5474)
  line L37 (40.32, 35.9874) -> (-2.5274, 35.9874) construction
  line L38 (10.71, 17.0349) -> (15.79, 17.0349)
  line L39 (15.79, 17.0349) -> (15.79, 18.8349)
  line L40 (15.79, 18.8349) -> (10.71, 18.8349)
  line L41 (10.71, 18.8349) -> (10.71, 17.0349)
  line L42 (26.75, 17.0349) -> (31.83, 17.0349)
  line L43 (31.83, 17.0349) -> (31.83, 18.8349)
  line L44 (31.83, 18.8349) -> (26.75, 18.8349)
  line L45 (26.75, 18.8349) -> (26.75, 17.0349)
  line L46 (35.97, 25.4274) -> (37.77, 25.4274)
  line L47 (37.77, 25.4274) -> (37.77, 30.5074)
  line L48 (37.77, 30.5074) -> (35.97, 30.5074)
  line L49 (35.97, 30.5074) -> (35.97, 25.4274)
  point P0 (-19.215, 23.2874)
  dimension "d194" = 5.08
  dimension "d195" = 0.4
  dimension "d196" = 0.4
  dimension "d197" = 5.08
  dimension "d198" = 5.08
  dimension "d199" = 0.4
  constraints: 50 end point, 12 symmetric about line, 6 parallel, 6 point on line, 4 perpendicular, 3 horizontal, 1 midpoint
  measures "d194" distance from line of L25.end L28
  measures "d195" distance from line of L25.end L6
  measures "d196" distance between parallel lines of L24 L32
  measures "d197" distance between parallel lines of L32 L30
  measures "d198" distance of L33.end L34.end
  measures "d199" distance between parallel lines of L21 L35
extrude "nubs" add sketch "Sketch28" along normal blind 1.8 contours L0 L35 L4 L33 | L32 L1 L30 L3 | L3 L28 L2 L26 | L48 L47 L46 L4 | L41 L40 L39 L38 | L45 L44 L43 L42
chamfer "nubchamfer" distance 1.8 angle 45 6 edges at (51.045, 62.1271, 5.3525) (29.925, 62.1271, 5.3525) (56.085, 62.1271, -2.14) (56.085, 62.1271, -23.26) (51.045, 62.1271, -30.7525) (29.925, 62.1271, -30.7525)
fillet "nubfillet" radius 1.5 18 edges at (35.005, 60.3271, 5.3525) (35.005, 62.1271, 5.3525) (45.965, 62.1271, 5.3525) (45.965, 60.3271, 5.3525) (56.085, 62.1271, -7.22) (56.085, 60.3271, -7.22) (56.085, 60.3271, -18.18) (56.085, 62.1271, -18.18) (45.965, 60.3271, -30.7525) (45.965, 62.1271, -30.7525) (35.005, 60.3271, -30.7525) (35.005, 62.1271, -30.7525) (56.085, 62.1271, -3.9399) (56.085, 62.1271, -21.4601) (49.2451, 62.1271, -30.7525) (31.7249, 62.1271, -30.7525) (49.2451, 62.1271, 5.3525) (31.7249, 62.1271, 5.3525)
equation "\"d1\" = d0"
equation "\"d7\" = d9 + d6 + d2"
equation "\"d10\" = d9 + d6 + d2"
equation "\"d12\" = d0"
equation "\"d14\" = d0"
equation "\"d9\" = 0.656244"
equation "\"d6\" = 2.296256"
equation "\"d2\" = 1.5"
body "Solid1"
